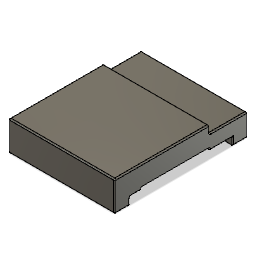
Tail Stock Base (Autodesk Fusion 360 design; units mm, degrees)
Autodesk Fusion 360 part; units mm, degrees
sketch "Sketch1" plane through (0, 0, 0) normal (0, 1, 0) x (1, 0, 0)
  line L0 (0, 0) -> (-88.9, 0)
  line L1 (-88.9, 0) -> (-88.9, -111.125)
  line L2 (-88.9, -111.125) -> (0, -111.125)
  line L3 (0, -111.125) -> (0, 0)
  line L4 (0, -12.7) -> (-88.9, -12.7)
  line L5 (0, -31.75) -> (-88.9, -31.75)
  line L6 (0, -88.9) -> (-88.9, -88.9)
  line L7 (0, -98.425) -> (-88.9, -98.425)
  dimension "d1" = 88.9
  dimension "d2" = 111.125
  dimension "d3" = 12.7
  dimension "d5" = 19.05
  dimension "d6" = 12.7
  dimension "d7" = 9.525
  constraint horizontal L0
  constraint vertical L1
  constraint horizontal L2
  constraint vertical L3
  constraint coincident L0.start L3.end
  constraint coincident L3 L4.start
  constraint coincident L1 L4.end
  constraint perpendicular L1 L4
  constraint coincident L3 L5.start
  constraint coincident L1 L5.end
  constraint perpendicular L1 L5
  constraint coincident L3 L6.start
  constraint coincident L1 L6.end
  constraint perpendicular L1 L6
  constraint coincident L3 L7.start
  constraint coincident L1 L7.end
  constraint perpendicular L1 L7
  measures "d1" distance of L0.start L0.end
  measures "d2" distance of L0.start L2.end
  measures "d3" distance of L0 L4
  measures "d5" distance of L4 L5
  measures "d6" distance of L2 L7
  measures "d7" distance of L6 L7
extrude "Extrude1" add sketch "Sketch1" along normal blind 25.4 contours L1 L3 L5 L6 | L1 L3 L6 L7 | L1 L2 L3 L7
extrude "Extrude2" add sketch "Sketch1" along normal blind 19.05 contours L0 L1 L3 L4 | L1 L3 L4 L5
extrude "Extrude3" cut sketch "Sketch1" along normal blind 6.35 contours L1 L3 L4 L5 | L1 L3 L6 L7
extrude "Extrude4" cut sketch "Sketch1" along normal blind 7.9375 contours L1 L3 L5 L6
fillet "Fillet1" radius 1 13 edges at (-44.45, 6.35, 98.425) (-44.45, 6.35, 88.9) (-44.45, 7.9375, 88.9) (-44.45, 7.9375, 31.75) (-44.45, 6.35, 31.75) (-44.45, 0, 12.7) (-44.45, 0, 98.425) (-44.45, 0, 0) (-44.45, 19.05, 0) (-44.45, 19.05, 31.75) (-44.45, 25.4, 31.75) (-44.45, 25.4, 111.125) (-44.45, 0, 111.125)
fillet "Fillet2" radius 1 2 faces at (0, 19.5792, 76.9393) (-88.9, 19.5792, 76.9393)
equation "d2 = 4 3/8\""
equation "d7 = 3 in / 8"
equation "d14 = 0.25 in + 1\" / 16"
